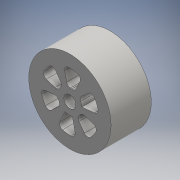
# Autodesk Inventor part: rin
Saved by Autodesk Inventor 2016 SP1 (Build 200210100, 210)
## iProperties
Created: 2016-10-02
Part Number: rin
Material: Generic
Document SubType Name: Modeling
Designer: CASA
Density: 1 g/cm^3
Appearance: Default
Author: CASA
Autodesk Inventor part; units mm, degrees
ref_plane "YZ Plane" through (0, 0, 0) normal (1, 0, 0) x (0, 1, 0)
ref_plane "XZ Plane" through (0, 0, 0) normal (0, 1, 0) x (-1, 0, 0)
ref_plane "XY Plane" through (0, 0, 0) normal (0, 0, 1) x (1, 0, 0)
sketch "Sketch1" plane through (0, 0, 0) normal (0, 1, 0) x (-1, 0, 0)
  circle A0 centre (0, 0) radius 10.25
  circle A1 centre (0, 0) radius 3
  line L0 (0, 0) -> (0, 7.25)
  line L1 (0, 0) -> (-4.2614, 5.8654)
  line L2 (0, 0) -> (-6.8952, 2.2404)
  line L3 (0, 0) -> (-6.8952, -2.2404)
  line L4 (0, 0) -> (-4.2614, -5.8654)
  line L5 (0, 0) -> (0, -7.25)
  line L6 (0, 0) -> (4.2614, -5.8654)
  line L7 (0, 0) -> (6.8952, -2.2404)
  line L8 (0, 0) -> (6.8952, 2.2404)
  line L9 (0, 0) -> (4.2614, 5.8654)
  arc A2 (4.2614, 5.8654) -> (0, 7.25) centre (0, 0) ccw
  arc A3 (-4.2614, 5.8654) -> (-6.8952, 2.2404) centre (0, 0) ccw
  arc A4 (-6.8952, -2.2404) -> (-4.2614, -5.8654) centre (0, 0) ccw
  arc A5 (0, -7.25) -> (4.2614, -5.8654) centre (0, 0) ccw
  arc A6 (6.8952, -2.2404) -> (6.8952, 2.2404) centre (0, 0) ccw
  arc A7 (4.2614, 5.8654) -> (0, 7.25) centre (0, 0) ccw
  arc A8 (6.8952, -2.2404) -> (6.8952, 2.2404) centre (0, 0) ccw
  arc A9 (0, -7.25) -> (4.2614, -5.8654) centre (0, 0) ccw
  arc A10 (-6.8952, -2.2404) -> (-4.2614, -5.8654) centre (0, 0) ccw
  arc A11 (-4.2614, 5.8654) -> (-6.8952, 2.2404) centre (0, 0) ccw
  circle A12 centre (0, 0) radius 3
  dimension "d0" = 20.5
  dimension "d2" = 6
  dimension "d5" = 360
  constraints: 20 end point, 20 point on circle, 13 centre point, 7 coincident, 2 point on line, 1 vertical, 31 other
  measures "d0" diameter of A0
  measures "d2" diameter of A1
extrude "Extrusion1" add sketch "Sketch1" along normal blind 10 contours A0 | A1 L7 L8 | A1 L8 A6 L7 | L8 L9 A1 | A1 L6 L7 | L9 L0 A1 | A1 L0 A2 L9 | L1 A1 L0 | L2 A1 L1 | L3 A1 L2 | L4 A1 L3 | L5 A1 L4 | L6 A1 L5 | L6 A5 L5 A1 | A1 L2 A3 L1
sketch "Sketch2" plane through (0, 10, 0) normal (0, 1, 0) x (1, 0, 0)
  point P0 (0, 0)
sketch "Sketch3" plane through (0, 10, 0) normal (0, 1, 0) x (1, 0, 0)
  arc A0 (2.8532, 0.9271) -> (1.7634, 2.4271) centre (0, 0) ccw
  line L0 (1.7634, 2.4271) -> (4.2614, 5.8654)
  arc A1 (6.8952, 2.2404) -> (4.2614, 5.8654) centre (0, 0) ccw
  line L1 (6.8952, 2.2404) -> (2.8532, 0.9271)
  line L2 (-1.2202, 2.7406) -> (-2.9488, 6.6232)
  arc A2 (0.6237, 2.9344) -> (-1.2202, 2.7406) centre (0, 0) ccw
  line L3 (1.5074, 7.0916) -> (0.6237, 2.9344)
  arc A3 (1.5074, 7.0916) -> (-2.9488, 6.6232) centre (0, 0) ccw
  line L4 (-2.9836, 0.3136) -> (-7.2103, 0.7578)
  arc A4 (-2.2294, 2.0074) -> (-2.9836, 0.3136) centre (0, 0) ccw
  line L5 (-5.3878, 4.8512) -> (-2.2294, 2.0074)
  arc A5 (-5.3878, 4.8512) -> (-7.2103, 0.7578) centre (0, 0) ccw
  line L6 (-1.7634, -2.4271) -> (-4.2614, -5.8654)
  arc A6 (-2.8532, -0.9271) -> (-1.7634, -2.4271) centre (0, 0) ccw
  line L7 (-6.8952, -2.2404) -> (-2.8532, -0.9271)
  arc A7 (-6.8952, -2.2404) -> (-4.2614, -5.8654) centre (0, 0) ccw
  line L8 (1.2202, -2.7406) -> (2.9488, -6.6232)
  arc A8 (-0.6237, -2.9344) -> (1.2202, -2.7406) centre (0, 0) ccw
  line L9 (-1.5074, -7.0916) -> (-0.6237, -2.9344)
  arc A9 (-1.5074, -7.0916) -> (2.9488, -6.6232) centre (0, 0) ccw
  line L10 (2.9836, -0.3136) -> (7.2103, -0.7578)
  arc A10 (2.2294, -2.0074) -> (2.9836, -0.3136) centre (0, 0) ccw
  line L11 (5.3878, -4.8512) -> (2.2294, -2.0074)
  arc A11 (5.3878, -4.8512) -> (7.2103, -0.7578) centre (0, 0) ccw
  dimension "d11" = 360
  constraints: 24 centre point, 24 end point, 24 point on circle, 61 other
extrude "Extrusion2" cut sketch "Sketch3" against normal blind 10 contours L2 A3 L3 A2 | L4 A5 L5 A4 | L6 A7 L7 A6 | L8 A9 L9 A8 | L10 A11 L11 A10
fillet "Fillet1" radius 1 21 edges at (-6.8952, 5, 2.2404) (-7.2103, 5, -0.7578) (-2.9488, 5, -6.6232) (1.7634, 5, -2.4271) (2.2294, 5, 2.0074) (-1.5074, 5, 7.0916) (2.8532, 5, -0.9271) (2.9488, 5, 6.6232) (-2.9836, 5, -0.3136) (6.8952, 5, -2.2404) (5.3878, 5, 4.8512) (7.2103, 5, 0.7578) (1.5074, 5, -7.0916) (-5.3878, 5, -4.8512) (4.2614, 5, -5.8654) (-0.6237, 5, 2.9344) (1.2202, 5, 2.7406) (-2.8532, 5, 0.9271) (-4.2614, 5, 5.8654) (-1.7634, 5, 2.4271) (-2.2294, 5, -2.0074)
sketch "Sketch4" plane through (0, 10, 0) normal (0, 1, 0) x (1, 0, 0)
  circle A0 centre (0, 0) radius 1.5
  dimension "d16" = 3
  constraints: 1 centre point, 1 coincident
  measures "d16" diameter of A0
extrude "Extrusion3" cut sketch "Sketch4" against normal blind 10
body "Solid1"
